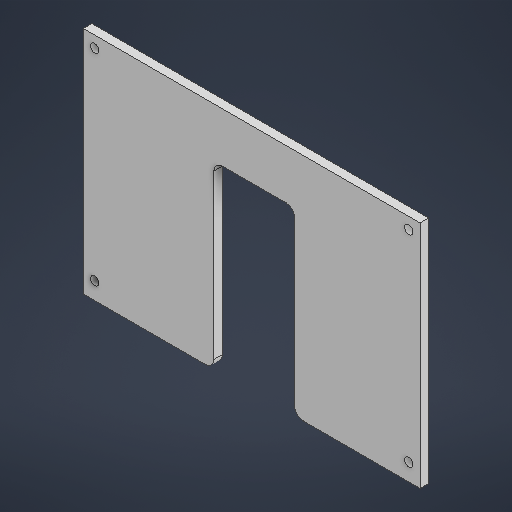
# Autodesk Inventor part: 底板
Saved by Autodesk Inventor 2025 (Build 290162000, 162)
## iProperties
Created: 2026-04-20
Part Number: 底板
Material: 常规
Document SubType Name: Modeling
Designer: XH
Density: 1 g/cm^3
Appearance: 默认
Author: XH
Autodesk Inventor part; units mm, degrees
ref_plane "YZ Plane" through (0, 0, 0) normal (1, 0, 0) x (0, 1, 0)
ref_plane "XZ Plane" through (0, 0, 0) normal (0, 1, 0) x (-1, 0, 0)
ref_plane "XY Plane" through (0, 0, 0) normal (0, 0, 1) x (1, 0, 0)
sketch "草图1" plane through (0, 0, 0) normal (0, 0, 1) x (1, 0, 0)
  line L0 (-63.2473, -48.717) -> (-63.2473, 31.8554) projected
  line L1 (56.7527, -48.717) -> (56.7527, -8.4207) projected
  line L2 (56.7527, -48.717) -> (-64.2305, -48.717)
  line L3 (-64.2305, -48.717) -> (-64.2305, 31.8463)
  line L4 (-64.2305, 31.8463) -> (56.7527, 31.8463)
  line L5 (56.7527, 31.8463) -> (56.7527, -48.717)
  line L6 (53.7527, -48.717) -> (53.7527, -8.4207) projected
  line L7 (-60.2473, -48.717) -> (-60.2473, 31.8554) projected
  line L8 (-59.7473, -48.717) -> (53.2527, -48.717)
  line L9 (53.2527, -48.717) -> (53.2527, 31.8463)
  line L10 (53.2527, 31.8463) -> (-59.7473, 31.8463)
  line L11 (-59.7473, 31.8463) -> (-59.7473, -48.717)
  point P0 (-59.7473, 31.8463)
  point P1 (53.2527, -48.717)
  dimension "d3" = 0.5
  dimension "d4" = 0.5
  constraints: 16 end point, 4 parallel, 2 horizontal, 2 perpendicular, 2 point on line
  measures "d3" distance from line of L6 L8.end
  measures "d4" distance of L7.start L8.start
extrude "拉伸1" add sketch "草图1" along normal blind 3 contours L11 L4 L9 L2
sketch "草图2" plane through (0, 0, 3) normal (0, 0, 1) x (1, 0, 0)
  circle A0 centre (-6.9652, -43.4115) radius 1.5 projected
  circle A1 centre (-6.9652, -5.4115) radius 1.5 projected
  circle A2 centre (39.5219, -43.4293) radius 1.5 projected
  circle A3 centre (39.5219, -5.4293) radius 1.5 projected
  point P0 (0, 0)
extrude "拉伸2" cut sketch "草图2" against normal blind 10
sketch "草图3" plane through (0, 0, 0) normal (0, 0, -1) x (-1, 0, 0)
  circle A0 centre (55.7473, -42.717) radius 1.5 projected
  circle A1 centre (55.7473, 27.8554) radius 1.5 projected
  circle A2 centre (-51.2527, -42.717) radius 1.5 projected
  circle A3 centre (-49.7527, 27.8554) radius 1.5 projected
extrude "拉伸3" cut sketch "草图3" against normal blind 10
sketch "草图4" plane through (0, 0, 0) normal (0, 0, -1) x (-1, 0, 0)
  circle A0 centre (22.7409, -46.1295) radius 1.5875 projected
  circle A1 centre (46.0659, -46.1295) radius 1.5875 projected
  circle A2 centre (46.0659, -0.092) radius 1.5875 projected
  circle A3 centre (22.7409, -0.092) radius 1.5875 projected
  circle A4 centre (46.0659, -46.1295) radius 2.0875
  circle A5 centre (22.7409, -46.1295) radius 2.0875
  circle A6 centre (22.7409, -0.092) radius 2.0875
  circle A7 centre (46.0659, -0.092) radius 2.0875
  point P0 (0, 0)
  dimension "d11" = 0.5
  dimension "d12" = 0.5
  dimension "d13" = 0.5
  dimension "d14" = 0.5
  constraints: 4 centre point
  measures "d11" radial gap between concentric circles of A1 A4
  measures "d12" radial gap between concentric circles of A0 A5
  measures "d13" radial gap between concentric circles of A3 A6
  measures "d14" radial gap between concentric circles of A2 A7
extrude "拉伸4" cut sketch "草图4" against normal blind 10 contours A0 | A1 | A2 | A3 | A4 | A5 | A6 | A7
sketch "草图5" plane through (0, 0, 3) normal (0, 0, 1) x (1, 0, 0)
  circle A0 centre (12.9757, -15.4117) radius 1.5 projected
  circle A1 centre (12.9757, 22.5884) radius 1.5 projected
  point P0 (0, 0)
extrude "拉伸5" cut sketch "草图5" against normal blind 10
sketch "草图6" plane through (0, 0, 0) normal (0, 0, -1) x (-1, 0, 0)
  circle A0 centre (-12.9757, -15.4117) radius 1.5 projected
  circle A1 centre (-12.9757, 22.5884) radius 1.5 projected
  circle A2 centre (46.0659, -0.092) radius 2.0875 projected
  circle A3 centre (46.0659, -46.1295) radius 2.0875 projected
  circle A4 centre (22.7409, -46.1295) radius 2.0875 projected
  circle A5 centre (22.7409, -0.092) radius 2.0875 projected
  circle A6 centre (55.7473, 27.8554) radius 1.5 projected
  circle A7 centre (-51.2527, -42.717) radius 1.5 projected
  circle A8 centre (55.7473, -42.717) radius 1.5 projected
  circle A9 centre (-49.7527, 27.8554) radius 1.5 projected
  circle A10 centre (6.9652, -5.4115) radius 1.5 projected
  circle A11 centre (-39.5219, -5.4293) radius 1.5 projected
  circle A12 centre (6.9652, -43.4115) radius 1.5 projected
  circle A13 centre (-39.5219, -43.4293) radius 1.5 projected
  line L0 (59.7473, -48.717) -> (-53.2527, -48.717) projected
  line L1 (59.7473, 31.8463) -> (59.7473, -48.717) projected
  line L2 (-53.2527, 31.8463) -> (59.7473, 31.8463) projected
  line L3 (-53.2527, -48.717) -> (-53.2527, 31.8463) projected
  point P0 (0, 0)
extrude "拉伸6" add sketch "草图6" against normal up to surface (3 mm away) contours A0 | A1 | A2 | A3 | A4 | A5 | A10 | A11 | A12 | A13
sketch "草图7" plane through (0, 0, 3) normal (0, 0, 1) x (1, 0, 0)
  line L0 (-14.0154, 14.4424) -> (29.279, 14.4424)
  line L1 (29.279, 14.4424) -> (29.279, -48.717)
  line L2 (29.279, -48.717) -> (-14.0154, -48.717)
  line L3 (-14.0154, -48.717) -> (-14.0154, 14.4424)
  line L4 (-59.7473, -48.717) -> (53.2527, -48.717) projected
  line L5 (2.5579, 11.4424) -> (-21.3741, 11.4424) projected
  point P0 (0, 0)
  dimension "d19" = 3
  constraints: 8 end point, 2 parallel, 1 collinear, 1 horizontal, 1 perpendicular
  measures "d19" distance between parallel lines of L0 L5
extrude "拉伸7" cut sketch "草图7" against normal blind 10
move faces "移动1" translate (-15, 0, 0) faces at (29.279, -27.6639, 1)
move faces "移动2" translate (4, 0, 0) faces at (53.2527, -21.8626, 1)
delete faces "删除1" heal yes whole lump no faces at (48.2721, 27.6147, 1) (49.7721, -42.9576, 1) (-57.2279, 27.6147, 1) (-55.6869, -41.2182, 2)
sketch "草图8" plane through (57.2527, 31.8463, 0) normal (0, 0, -1) x (-1, 0, 0)
  circle A0 centre (113, -3.9909) radius 1.5 projected
  point P0 (57.2527, -31.8463)
extrude "拉伸8" cut sketch "草图8" against normal blind 10
move faces "移动3" translate (1, 0, 0) faces at (57.2527, -21.8626, 1)
sketch "草图9" plane through (-14.0154, -48.717, 0) normal (0, 0, -1) x (-1, 0, 0)
  circle A0 centre (41.7319, 6) radius 1.5 projected
  point P0 (-14.0154, 48.717)
extrude "拉伸9" cut sketch "草图9" against normal blind 10
sketch "草图10" plane through (-14.0154, -48.717, 0) normal (0, 0, -1) x (-1, 0, 0)
  circle A0 centre (-68.2681, 6) radius 1.5 projected
  point P0 (-14.0154, 48.717)
extrude "拉伸10" cut sketch "草图10" against normal blind 10
sketch "草图11" plane through (-14.0154, -48.717, 0) normal (0, 0, -1) x (-1, 0, 0)
  circle A0 centre (-68.2681, 76.5724) radius 1.5 projected
  point P0 (-14.0154, 48.717)
extrude "拉伸11" cut sketch "草图11" against normal blind 10
fillet "圆角1" radius 3 4 edges at (-14.0154, -48.717, 1.5) (14.279, -48.717, 1.5) (-14.0154, 14.4424, 1.5) (14.279, 14.4424, 1.5)
